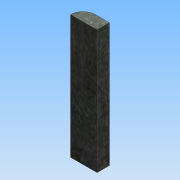
# Autodesk Inventor part: Paper-holder-clip
Saved by Autodesk Inventor 2016 (Build 200138000, 138)
## iProperties
Created: 2015-10-22
Part Number: Paper-holder-clip
Material: Steel
Document SubType Name: Modeling
Designer: Openlab
Density: 7.85 g/cm^3
Appearance: Plate
Author: Openlab
Autodesk Inventor part; units mm, degrees
ref_plane "YZ Plane" through (0, 0, 0) normal (1, 0, 0) x (0, 1, 0)
ref_plane "XZ Plane" through (0, 0, 0) normal (0, 1, 0) x (-1, 0, 0)
ref_plane "XY Plane" through (0, 0, 0) normal (0, 0, 1) x (1, 0, 0)
sketch "Sketch1" plane through (0, 0, 0) normal (0, 1, 0) x (-1, 0, 0)
  line L0 (24.6138, 28.8821) -> (9.6138, 28.8821)
  line L1 (9.6138, 28.8821) -> (9.6138, -41.1179)
  line L2 (9.6138, -41.1179) -> (24.6138, -41.1179)
  line L3 (24.6138, -41.1179) -> (24.6138, 28.8821)
  point P0 (0, 0)
  dimension "d0" = 70
  dimension "d1" = 15
  constraints: 8 end point, 2 parallel, 1 horizontal, 1 perpendicular
  measures "d0" distance of L2.end L0.start
  measures "d1" distance of L0.start L0.end
extrude "Extrusion1" add sketch "Sketch1" along normal blind 7
fillet "Fillet1" radius 7 1 edges at (-24.6138, 7, -6.1179)
body "Solid1"
